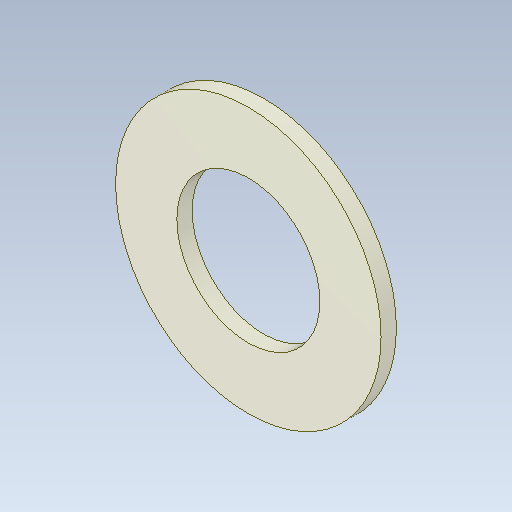
# Autodesk Inventor part: PTFE_Anlaufscheibe
Saved by Autodesk Inventor 2021.4 (Build 254397000, 397)
## iProperties
Created: 2022-07-11
Part Number: PTFE_Anlaufscheibe
Material: Polytetrafluoroethylene
Document SubType Name: Modeling
Designer: alexw
Mass: 1.14228 g
Surface Area: 9.42478 cm^2
Volume: 0.565487 cm^3
Density: 2.02 g/cm^3
Appearance: Smooth - Ivory
Author: alexw
Autodesk Inventor part; units mm, degrees
ref_plane "YZ Plane" through (0, 0, 0) normal (1, 0, 0) x (0, 1, 0)
ref_plane "XZ Plane" through (0, 0, 0) normal (0, 1, 0) x (-1, 0, 0)
ref_plane "XY Plane" through (0, 0, 0) normal (0, 0, 1) x (1, 0, 0)
sketch "Sketch1" plane through (0, 0, 0) normal (0, 0, 1) x (1, 0, 0)
  circle A0 centre (0, 0) radius 13
  circle A1 centre (0, 0) radius 7
  dimension "d0" = 26
  dimension "d1" = 14
  constraints: 2 centre point, 2 coincident
  measures "d0" diameter of A0
  measures "d1" diameter of A1
extrude "Extrusion1" add sketch "Sketch1" along normal blind 1.5
body "Solid1"
